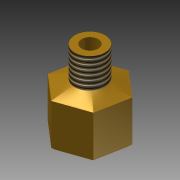
# Autodesk Inventor part: 222P-4-2
Saved by Autodesk Inventor 2011 (Build 150239000, 239)
## iProperties
Category: Pneumatics
Shininess: 64.0
Length Units: 11269
Angle Units: 11279
Time Units: 11290
Mass Units: 11283
Length Display Precision: 3
Angle Display Precision: 2
Compacted: True
Document SubType Name: Modeling
Created: 2005-01-08
Manufacturer: Standard
Standards Organization: Custom
Description: Adapter 1/4 in Female to 1/8 in Male
Vendor: Parker
Project: FIRST
Part Number: 222P-4-2
Density: 1 g/cm^3
Density: 0.0
Volumn: 0.0
Area: 0.0
PropertySet Name: Model Information
Control State: 0
Master: False
Checked Out: False
Title: Adapter 1/4 in Female to 1/8 in Male
Author: Autodesk, Inc.
Autodesk Inventor part; units mm, degrees
ref_plane "YZ Plane" through (0, 0, 0) normal (1, 0, 0) x (0, 1, 0)
ref_plane "XZ Plane" through (0, 0, 0) normal (0, 1, 0) x (-1, 0, 0)
sketch "Sketch1" plane through (0, 0, 0) normal (0, 0, 1) x (1, 0, 0)
  line L0 (2.0695, 10.8021) -> (10.3896, 3.6088)
  line L1 (10.3896, 3.6088) -> (8.3201, -7.1932)
  line L2 (8.3201, -7.1932) -> (-2.0695, -10.8021)
  line L3 (-2.0695, -10.8021) -> (-10.3896, -3.6088)
  line L4 (-10.3896, -3.6088) -> (-8.3201, 7.1932)
  line L5 (-8.3201, 7.1932) -> (2.0695, 10.8021)
  point P0 (0, 0)
  point P1 (0, 0)
  dimension "d0" = 19.05
  constraints: 12 end point, 1 coincident, 11 other
  measures "d0" distance between parallel lines of L2 L5
extrude "Extrusion1" add sketch "Sketch1" along normal blind 14.478
ref_plane "Work Plane1" through (0, 0, 16.51) normal (0, 0, 1) x (1, 0, 0)
sketch "Sketch2" plane through (0, 0, 16.51) normal (0, 0, 1) x (1, 0, 0)
  circle A0 centre (0, 0) radius 5
  dimension "d4" = 10
  constraints: 1 centre point, 1 coincident
  measures "d4" diameter of A0
sketch "Sketch3" plane through (0, 0, 14.478) normal (0, 0, 1) x (1, 0, 0)
  line L0 (10.3896, 3.6088) -> (8.3201, -7.1932) projected
  line L1 (2.0695, 10.8021) -> (10.3896, 3.6088) projected
  line L2 (-8.3201, 7.1932) -> (2.0695, 10.8021) projected
  line L3 (-10.3896, -3.6088) -> (-8.3201, 7.1932) projected
  line L4 (-2.0695, -10.8021) -> (-10.3896, -3.6088) projected
  line L5 (8.3201, -7.1932) -> (-2.0695, -10.8021) projected
loft "Loft1" add profiles "Sketch3", "Sketch2"
extrude "Extrusion2" add sketch "Sketch2" along normal blind 10
sketch "Sketch4" plane through (0, 0, 0) normal (0, 0, -1) x (-1, 0, 0)
  circle A0 centre (0, 0) radius 5.75
  dimension "d11" = 11.5
  constraints: 1 centre point
  measures "d11" diameter of A0
extrude "Extrusion3" cut sketch "Sketch4" against normal blind 11.75
sketch "Sketch5" plane through (0, 0, 11.75) normal (0, 0, -1) x (-1, 0, 0)
  circle A0 centre (0, 0) radius 2.75
  dimension "d14" = 5.5
  constraints: 1 centre point
  measures "d14" diameter of A0
extrude "Extrusion4" cut sketch "Sketch5" against normal blind 19
thread "Thread1" size "M10x1.5" class "6g" standard "ANSI Metric M Profile" full length
thread "Thread2" size "M12x1.75" class "6H" standard "ANSI Metric M Profile" full length
chamfer "Chamfer1" distance 1 angle 45 7 edges at (9.3549, -1.7922, 0) (6.2295, 7.2055, 0) (-3.1253, 8.9977, 0) (-9.3549, 1.7922, 0) (-6.2295, -7.2055, 0) (3.1253, -8.9977, 0) (5.75, 0, 0)
body "Solid1"
